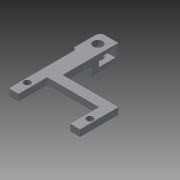
# Autodesk Inventor part: ServoBracket
Saved by Autodesk Inventor 2014 SP1 (Build 180222100, 222)
## iProperties
Created: 2017-02-13
Part Number: ServoBracket
Material: Generic
Document SubType Name: Modeling
Designer: danielsikar
Density: 1 g/cm^3
Appearance: Default
Author: danielsikar
Autodesk Inventor part; units mm, degrees
ref_plane "YZ Plane" through (0, 0, 0) normal (1, 0, 0) x (0, 1, 0)
ref_plane "XZ Plane" through (0, 0, 0) normal (0, 1, 0) x (-1, 0, 0)
sketch "Sketch1" plane through (0, 0, 0) normal (0, 0, 1) x (1, 0, 0)
  line L0 (22.8, 0) -> (0, 0) projected
  line L1 (22.8, 12.5) -> (22.8, 0) projected
  line L2 (0, 12.5) -> (22.8, 12.5) projected
  line L3 (0, 0) -> (0, 12.5) projected
  arc A0 (-3.7, 5.65) -> (-3.7, 6.85) centre (-2.9, 6.25) ccw projected
  arc A1 (26.5, 6.85) -> (26.5, 5.65) centre (25.7, 6.25) ccw projected
  line L4 (23.2, 12.9) -> (23.2, -0.4)
  line L5 (23.2, -0.4) -> (-0.4, -0.4)
  line L6 (-0.4, -0.4) -> (-0.4, 12.9)
  line L7 (-0.4, 12.9) -> (23.2, 12.9)
  line L8 (27.6, 6.85) -> (27.6, 12.5) construction
  line L9 (27.629, -4.829) -> (27.629, 17.329)
  line L10 (27.629, 17.329) -> (-4.829, 17.329)
  line L11 (-4.829, 17.329) -> (-4.829, -4.829)
  line L12 (-4.829, -4.829) -> (27.629, -4.829)
  arc A2 (-4.1, 5.35) -> (-4.1, 7.15) centre (-2.9, 6.25) ccw
  arc A3 (26.9, 7.15) -> (26.9, 5.35) centre (25.7, 6.25) ccw
  circle A4 centre (-2.9, 6.25) radius 1.5
  circle A5 centre (25.7, 6.25) radius 1.5
  dimension "d0" = 0.4
  dimension "d1" = 0.5
  dimension "d2" = 0.5
  constraints: 16 end point, 4 centre point, 4 point on circle, 2 coincident, 2 concentric, 6 other
  measures "d0" distance between parallel lines of L2 L7
  measures "d1" radial gap between concentric circles of A2 A0
  measures "d2" radial gap between concentric circles of A1 A3
extrude "Extrusion1" add sketch "Sketch1" along normal blind 3 contours L12 L11 L10 L9
sketch "Sketch2" plane through (-4.829, -4.829, 0) normal (0, -1, 0) x (1, 0, 0)
  line L0 (0, 0) -> (32.458, 0) projected
  line L1 (32.458, 0) -> (32.458, 3) projected
  line L2 (0, 3) -> (32.458, 3) projected
  line L3 (0, 0) -> (0, 3) projected
  point P0 (4.829, 0)
extrude "Extrusion2" cut sketch "Sketch2" against normal blind 4.6
sketch "Sketch3" plane through (-4.829, 17.329, 0) normal (0, 1, 0) x (1, 0, 0)
  line L0 (32.458, -3) -> (0, -3) projected
  line L1 (0, 0) -> (7, 0)
  line L2 (7, 0) -> (7, -3)
  line L3 (7, -3) -> (0, -3)
  line L4 (0, -3) -> (0, 0)
  point P0 (4.829, 0)
  dimension "d7" = 7
  constraints: 8 end point, 2 parallel, 1 horizontal, 1 perpendicular, 1 point on line
  measures "d7" distance of L2.end L3.end
ref_plane "Work Plane1" through (-4.1, 42.6608, -9.2) normal (0, 1, 0) x (0, 0, 1)
extrude "Extrusion3" add sketch "Sketch3" along normal up to surface (25.3318 mm away)
sketch "Sketch4" plane through (0, 0, 0) normal (0, 0, -1) x (-1, 0, 0)
  circle A0 centre (2.1, 37.6608) radius 2 projected
  line L0 (-1.9, 39.6608) -> (-1.9, 32.6608) projected
  line L1 (-6.3422, 39.6608) -> (-1.9, 39.6608) projected
  line L2 (-6.3422, 39.6608) -> (-6.3422, 42.6608) projected
  line L3 (-6.3422, 42.6608) -> (4.1, 42.6608) projected
  arc A1 (6.1, 40.6608) -> (4.1, 42.6608) centre (4.1, 40.6608) ccw projected
  line L4 (6.1, 32.6608) -> (6.1, 40.6608) projected
  line L5 (-1.9, 32.6608) -> (6.1, 32.6608) projected
  point P0 (0, 0)
extrude "Extrusion4" add sketch "Sketch4" along normal up to surface (4.2 mm away)
sketch "Sketch5" plane through (0, 0, 0) normal (0, 0, 1) x (1, 0, 0)
  line L0 (2.171, 39.6608) -> (2.171, 42.6608) projected
  line L1 (6.3422, 39.6608) -> (2.171, 39.6608) projected
  line L2 (6.3422, 42.6608) -> (6.3422, 39.6608) projected
  line L3 (2.171, 42.6608) -> (6.3422, 42.6608) projected
  point P0 (0, 0)
extrude "Extrusion5" cut sketch "Sketch5" against normal up to surface (4.2 mm away)
sketch "Sketch6" plane through (0, 0, 0) normal (0, 0, 1) x (1, 0, 0)
  line L0 (-4.829, 32.6608) -> (-4.829, 42.5232) projected
  arc A0 (-4.829, 42.5232) -> (-6.1, 40.6608) centre (-4.1, 40.6608) ccw projected
  line L1 (-6.1, 32.6608) -> (-6.1, 40.6608) projected
  line L2 (-4.829, 32.6608) -> (-6.1, 32.6608) projected
  point P0 (0, 0)
extrude "Extrusion6" add sketch "Sketch6" along normal up to surface (3 mm away)
sketch "Sketch7" plane through (1.9, 32.6608, 0) normal (1, 0, 0) x (0, 0, -1)
  line L0 (4.2, 0) -> (4.2, 7) projected
  line L1 (0, 7) -> (4.2, 7) projected
  line L2 (0, 0) -> (0, 7) projected
  line L3 (0, 0) -> (4.2, 0) projected
  point P0 (0, -32.6608)
extrude "Extrusion7" add sketch "Sketch7" along normal up to surface (0.271 mm away)
sketch "Sketch8" plane through (-6.1, 32.6608, -4.2) normal (-1, 0, 0) x (0, 0, 1)
  line L0 (2, 8.75) -> (5.5, 8.75)
  line L1 (5.5, 8.75) -> (5.5, 1.25)
  line L2 (5.5, 1.25) -> (2, 1.25)
  line L3 (2, 1.25) -> (2, 8.75)
  line L4 (0, 7) -> (0, 3) construction
  line L5 (0, 7) -> (0, 3) construction
  line L6 (4.2, 7) -> (4.2, 3) construction
  line L7 (4.2, 7) -> (0, 7) construction
  line L8 (4.2, 3) -> (0, 3) construction
  point P0 (4.2, -32.6608)
  dimension "d19" = 3.5
  dimension "d20" = 7.5
  dimension "d21" = 1.75
  dimension "d22" = 2
  constraints: 8 end point, 2 parallel, 1 horizontal, 1 perpendicular
  measures "d19" distance of L1.end L2.end
  measures "d20" distance of L0.end L1.end
  measures "d21" distance between parallel lines of L7 L0
  measures "d22" distance between parallel lines of L3 L5
extrude "Extrusion8" cut sketch "Sketch8" against normal through all
sketch "Sketch9" plane through (-6.1, 33.9108, 1.3) normal (0, 0, -1) x (-1, 0, 0)
  circle A0 centre (-4, 3.75) radius 2 projected
  circle A1 centre (-4, 3.75) radius 2.2
  point P0 (-6.1, -33.9108)
  dimension "d25" = 0.2
  constraints: 1 centre point
  measures "d25" radial gap between concentric circles of A1 A0
extrude "Extrusion9" cut sketch "Sketch9" along normal through all both and the other way through all contours A0 | A1
sketch "Sketch10" plane through (-4.829, 32.6608, 0) normal (0, -1, 0) x (1, 0, 0)
  line L0 (-1.271, -4.2) -> (7, -4.2) projected
  line L1 (7, -4.2) -> (7, 0) projected
  line L2 (0, 0) -> (7, 0) projected
  line L3 (0, 3) -> (0, 0) projected
  line L4 (0, 3) -> (-1.271, 3) projected
  line L5 (-1.271, 3) -> (-1.271, -4.2) projected
  point P0 (4.829, 0)
extrude "Extrusion10" add sketch "Sketch10" along normal blind 2
fillet "Fillet2" radius 1 2 edges at (-1.329, 30.6608, 0) (-4.829, 30.6608, 1.5)
body "Solid1"
